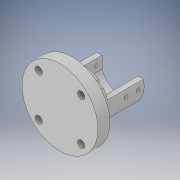
# Autodesk Inventor part: Part1_ur3Gripp
Saved by Autodesk Inventor 2019 (Build 230136000, 136)
## iProperties
Created: 2019-07-25
Part Number: Part1_ur3Gripp
Material: Generic
Document SubType Name: Modeling
Designer: romanp
Density: 1 g/cm^3
Appearance: Default
Author: romanp
Autodesk Inventor part; units mm, degrees
ref_plane "YZ Plane" through (0, 0, 0) normal (1, 0, 0) x (0, 1, 0)
ref_plane "XZ Plane" through (0, 0, 0) normal (0, 1, 0) x (-1, 0, 0)
ref_plane "XY Plane" through (0, 0, 0) normal (0, 0, 1) x (1, 0, 0)
sketch "Sketch1" plane through (0, 0, 0) normal (0, 0, 1) x (1, 0, 0)
  circle A0 centre (0, 0) radius 20
  circle A1 centre (-11.1369, 11.1369) radius 2.5
  circle A2 centre (11.1369, 11.1369) radius 2.5
  circle A3 centre (11.1369, -11.1369) radius 2.5
  circle A4 centre (-11.1369, -11.1369) radius 2.5
  dimension "d0" = 40
  dimension "d1" = 5
  dimension "d2" = 5
  dimension "d3" = 5
  dimension "d4" = 5
  constraints: 5 centre point, 2 coincident
  measures "d0" diameter of A0
  measures "d1" diameter of A1
  measures "d2" diameter of A2
  measures "d3" diameter of A3
  measures "d4" diameter of A4
extrude "Extrusion1" add sketch "Sketch1" against normal blind 10
sketch "Sketch2" plane through (0, 0, -10) normal (0, 0, -1) x (-1, 0, 0)
  line L0 (0, 0) -> (-20, 0)
  circle A0 centre (0, 0) radius 20 projected
  circle A1 centre (-11.1369, -11.1369) radius 2.5 projected
  circle A2 centre (11.1369, -11.1369) radius 2.5 projected
  line L1 (-11.1369, 0) -> (-11.1369, 5)
  line L2 (-11.1369, 5) -> (-19.3649, 5)
  line L3 (-11.1369, 0) -> (-11.1369, -5)
  line L4 (-11.1369, -5) -> (-19.3649, -5)
  line L5 (11.1369, -5) -> (19.3649, -5)
  line L6 (11.1369, 5) -> (19.3649, 5)
  line L7 (11.1369, -5) -> (11.1369, 5)
  line L8 (-11.1369, 5) -> (-11.1369, -5)
  arc A3 (-19.3649, 5) -> (-19.3649, -5) centre (0, 0) ccw
  arc A4 (19.3649, -5) -> (19.3649, 5) centre (0, 0) ccw
  dimension "d7" = 5
  dimension "d8" = 5
  constraints: 18 end point, 10 point on circle, 2 centre point, 2 perpendicular, 2 point on line, 1 concentric, 1 horizontal, 1 midpoint, 1 vertical
  measures "d7" distance of L1.start L1.end
  measures "d8" distance of L1.start L3.end
extrude "Extrusion2" add sketch "Sketch2" along normal blind 40 contours L3 L4 A0 L0 | L0 A0 L2 L1 | A0 L5 L7 L6
sketch "Sketch3" plane through (11.1369, -5, -10) normal (-1, 0, 0) x (0, 0, 1)
  circle A0 centre (-35, 5) radius 1.5
  circle A1 centre (-25, 5) radius 1.5
  point P0 (10, 5)
  point P1 (-40, 10)
  dimension "d22" = 3
  dimension "d23" = 3
  constraints: 2 centre point
  measures "d22" diameter of A0
  measures "d23" diameter of A1
extrude "Extrusion3" cut sketch "Sketch3" along normal mid plane 400
sketch "Sketch5" plane through (0, 0, -50) normal (0, 0, -1) x (-1, 0, 0)
  line L0 (-11.1369, -5) -> (-19.3649, -5) projected
  line L1 (11.1369, 5) -> (19.3649, 5) projected
  line L2 (19.3649, -5) -> (11.1369, -5) projected
  line L3 (-11.1369, 5) -> (-11.1369, -5) projected
  line L4 (-11.1369, 5) -> (-14.9999, 5)
  line L5 (-14.9999, 5) -> (-14.9999, -5)
  line L6 (-14.9999, -5) -> (-11.1369, -5)
  line L7 (-11.1369, -5) -> (-11.1369, 5)
  line L8 (11.1369, 5) -> (14.9999, 5)
  line L9 (14.9999, 5) -> (14.9999, -5)
  line L10 (14.9999, -5) -> (11.1369, -5)
  line L11 (11.1369, -5) -> (11.1369, 5)
  point P0 (0, 0)
  dimension "d26" = 3.863
  dimension "d27" = 3.863
  constraints: 16 end point, 4 parallel, 2 horizontal, 2 perpendicular, 2 point on line
  measures "d26" distance of L6.end L5.end
  measures "d27" distance of L9.end L10.end
extrude "Extrusion4" cut sketch "Sketch5" against normal blind 40
sketch "Sketch8" plane through (0, 0, 0) normal (0, 0, 1) x (1, 0, 0)
  circle A0 centre (0, 0) radius 31.5
  circle A1 centre (0, 0) radius 20
  dimension "d32" = 63
  constraints: 2 centre point, 1 coincident
  measures "d32" diameter of A0
extrude "Extrusion5" add sketch "Sketch8" against normal blind 10
sketch "Sketch9" plane through (0, 0, 0) normal (0, 0, 1) x (1, 0, 0)
  line L0 (0, 0) -> (44.6621, 0) construction
  line L1 (0, 0) -> (56.4016, 0) construction
  line L2 (0, 0) -> (52.8448, 0) construction
  line L3 (0, 0) -> (52.8448, 0) construction
  circle A0 centre (-17.6777, -17.6777) radius 3
  circle A1 centre (17.6777, -17.6777) radius 3
  circle A2 centre (17.6777, 17.6777) radius 3
  circle A3 centre (-17.6777, 17.6777) radius 3
  dimension "d40" = 6
  dimension "d41" = 6
  dimension "d42" = 6
  dimension "d43" = 6
  constraints: 8 end point, 4 centre point, 4 horizontal, 1 coincident
  measures "d40" diameter of A0
  measures "d41" diameter of A1
  measures "d42" diameter of A2
  measures "d43" diameter of A3
extrude "Extrusion6" cut sketch "Sketch9" against normal blind 10
sketch "Sketch10" plane through (0, 0, 0) normal (0, 0, 1) x (1, 0, 0)
  circle A0 centre (-11.1369, 11.1369) radius 2.5 projected
  circle A1 centre (-11.1369, 11.1369) radius 2.5
  circle A2 centre (11.1369, 11.1369) radius 2.5 projected
  circle A3 centre (11.1369, 11.1369) radius 2.5
  circle A4 centre (11.1369, -11.1369) radius 2.5 projected
  circle A5 centre (11.1369, -11.1369) radius 2.5
  circle A6 centre (-11.1369, -11.1369) radius 2.5 projected
  circle A7 centre (-11.1369, -11.1369) radius 2.5
  point P0 (0, 0)
  constraints: 4 centre point, 4 coincident
extrude "Extrusion7" add sketch "Sketch10" against normal blind 10
sketch "Sketch12" plane through (0, 0, -50) normal (0, 0, -1) x (-1, 0, 0)
  line L0 (-14.9999, -5) -> (-19.3649, -5) projected
  arc A0 (-19.3649, -5) -> (19.3649, -5) centre (0, 0) ccw
  arc A1 (-14.9999, -5) -> (14.9999, -5) centre (0, 0) ccw
  line L1 (14.9999, -5) -> (19.3649, -5) projected
  line L2 (-19.3649, -5) -> (-14.9999, -5)
  line L3 (14.9999, -5) -> (19.3649, -5)
  constraints: 5 point on circle, 4 end point, 2 centre point, 2 coincident, 2 collinear
extrude "Extrusion8" add sketch "Sketch12" against normal blind 40
sketch "Sketch13" plane through (0, 0, -10) normal (0, 0, -1) x (-1, 0, 0)
  circle A0 centre (-17.6777, -17.6777) radius 3 projected
  circle A1 centre (-17.6777, -17.6777) radius 6
  circle A2 centre (17.6777, -17.6777) radius 3 projected
  circle A3 centre (17.6777, -17.6777) radius 6
  point P0 (0, 0)
  dimension "d50" = 12
  dimension "d51" = 12
  constraints: 2 centre point, 2 coincident
  measures "d50" diameter of A1
  measures "d51" diameter of A3
extrude "Extrusion9" cut sketch "Sketch13" along normal blind 40
sketch "Sketch16" plane through (0, 0, -10) normal (0, 0, -1) x (-1, 0, 0)
  line L0 (19.3649, 5) -> (14.9999, 5) projected
  arc A0 (19.3649, 5) -> (-19.3649, 5) centre (0, 0) ccw
  arc A1 (14.9999, 5) -> (-14.9999, 5) centre (0, 0) ccw
  arc A2 (-19.3649, 5) -> (-16.0784, -11.8947) centre (0, 0) ccw projected
  line L1 (-19.3649, 5) -> (-14.9999, 5)
  line L2 (14.9999, 5) -> (19.3649, 5)
  constraints: 5 point on circle, 4 end point, 2 centre point, 2 coincident, 2 collinear
extrude "Extrusion10" add sketch "Sketch16" along normal blind 10
sketch "Sketch17" plane through (0, 0, -10) normal (0, 0, -1) x (-1, 0, 0)
  circle A0 centre (17.6777, 17.6777) radius 3 projected
  circle A1 centre (17.6777, 17.6777) radius 6
  circle A2 centre (-17.6777, 17.6777) radius 3 projected
  circle A3 centre (-17.6777, 17.6777) radius 6
  point P0 (0, 0)
  dimension "d58" = 12
  dimension "d59" = 12
  constraints: 2 centre point, 2 coincident
  measures "d58" diameter of A1
  measures "d59" diameter of A3
extrude "Extrusion11" cut sketch "Sketch17" along normal blind 15
body "Solid1"
